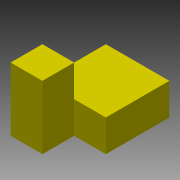
# Autodesk Inventor part: Part5
Saved by Autodesk Inventor 2013 (Build 170138000, 138)
## iProperties
Created: 2013-11-13
Part Number: Part5
Material: Generic
Document SubType Name: Modeling
Designer: s601298
Density: 1 g/cm^3
Mass: 41.4798 g
Surface Area: 87.0966 cm^2
Volume: 41.4798 cm^3
Author: s601298
Autodesk Inventor part; units mm, degrees
ref_plane "YZ Plane" through (0, 0, 0) normal (1, 0, 0) x (0, 1, 0)
ref_plane "XZ Plane" through (0, 0, 0) normal (0, 1, 0) x (-1, 0, 0)
ref_plane "XY Plane" through (0, 0, 0) normal (0, 0, 1) x (1, 0, 0)
sketch "Sketch1" plane through (0, 0, 0) normal (0, 1, 0) x (-1, 0, 0)
  line L0 (-14.1495, 10.3763) -> (23.9505, 10.3763)
  line L1 (23.9505, 10.3763) -> (23.9505, -27.7237)
  line L2 (23.9505, -27.7237) -> (-14.1495, -27.7237)
  line L3 (-14.1495, -27.7237) -> (-14.1495, 10.3763)
  point P0 (0, 0)
  dimension "d0" = 38.1
  dimension "d1" = 38.1
  constraints: 8 end point, 2 parallel, 1 horizontal, 1 perpendicular
  measures "d0" distance of L1.end L2.end
  measures "d1" distance of L0.end L1.end
extrude "Extrusion1" add sketch "Sketch1" along normal blind 19.05
sketch "Sketch2" plane through (-23.9505, 0, 10.3763) normal (0, 0, 1) x (1, 0, 0)
  line L0 (0, 0) -> (19.05, 0)
  line L1 (19.05, 0) -> (19.05, 38.1)
  line L2 (19.05, 38.1) -> (0, 38.1)
  line L3 (0, 38.1) -> (0, 0)
  point P0 (23.9505, 0)
  dimension "d4" = 19.05
  dimension "d5" = 38.1
  constraints: 8 end point, 2 parallel, 1 horizontal, 1 perpendicular
  measures "d4" distance of L2.end L1.end
  measures "d5" distance of L1.end L0.end
extrude "Extrusion2" add sketch "Sketch2" along normal blind 19.05
body "Solid1"
